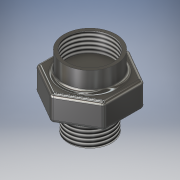
# Autodesk Inventor part: RKF 46-1M_NPT
Saved by Autodesk Inventor 2016 (Build 200138000, 138)
## iProperties
Created: 2016-03-26
Part Number: RKF 46-1M_NPT
Material: Brass, Soft Yellow
Document SubType Name: Modeling
Designer: agmle
Density: 8.47 g/cm^3
Appearance: Chrome - Polished
Author: agmle
Autodesk Inventor part; units mm, degrees
ref_plane "YZ Plane" through (0, 0, 0) normal (1, 0, 0) x (0, 1, 0)
ref_plane "XZ Plane" through (0, 0, 0) normal (0, 1, 0) x (-1, 0, 0)
ref_plane "XY Plane" through (0, 0, 0) normal (0, 0, 1) x (1, 0, 0)
sketch "Sketch1" plane through (0, 0, 0) normal (0, 1, 0) x (-1, 0, 0)
  line L0 (16.6553, -9.6469) -> (-0.0268, -19.2474)
  line L1 (-0.0268, -19.2474) -> (-16.6821, -9.6005)
  line L2 (-16.6821, -9.6005) -> (-16.6553, 9.6469)
  line L3 (-16.6553, 9.6469) -> (0.0268, 19.2474)
  line L4 (0.0268, 19.2474) -> (16.6821, 9.6005)
  line L5 (16.6821, 9.6005) -> (16.6553, -9.6469)
  point P0 (0, 0)
  point P1 (0, 0)
  dimension "d0" = 33.3375
  constraints: 12 end point, 1 coincident, 13 other
  measures "d0" distance between parallel lines of L2 L5
extrude "Extrusion1" add sketch "Sketch1" along normal blind 12.3031
sketch "Sketch2" plane through (0, 12.3031, 0) normal (0, 1, 0) x (1, 0, 0)
  circle A0 centre (0, 0) radius 12.7
  circle A1 centre (0, 0) radius 11.1125
  dimension "d3" = 25.4
  dimension "d16" = 22.225
  constraints: 2 centre point, 2 coincident
  measures "d3" diameter of A0
  measures "d16" diameter of A1
sketch "Sketch3" plane through (0, 0, 0) normal (0, -1, 0) x (1, 0, 0)
  circle A0 centre (0, 0) radius 10.541
  dimension "d8" = 21.082
  constraints: 1 centre point, 1 coincident
  measures "d8" diameter of A0
extrude "Extrusion3" add sketch "Sketch3" along normal blind 12.7
thread "Thread2" size "1/2" designation "1/2 - 14 NPT" standard "NPT" length 19.8628
fillet "Fillet1" radius 1.5875 6 edges at (16.6553, 6.1516, 9.6469) (-0.0268, 6.1516, 19.2474) (-16.6821, 6.1516, 9.6005) (16.6821, 6.1516, -9.6005) (0.0268, 6.1516, -19.2474) (-16.6553, 6.1516, -9.6469)
fillet "Fillet2" radius 1.5875 24 edges at (-16.4428, 12.3031, -9.5238) (-16.6687, 12.3031, -0.0232) (-16.4693, 12.3031, 9.478) (-8.3545, 12.3031, 14.4239) (-0.0265, 12.3031, 19.0018) (8.3143, 12.3031, 14.4471) (16.4428, 12.3031, 9.5238) (16.6687, 12.3031, 0.0232) (16.4693, 12.3031, -9.478) (8.3545, 12.3031, -14.4239) (0.0265, 12.3031, -19.0018) (-8.3143, 12.3031, -14.4471) (0.0265, 0, -19.0018) (8.3545, 0, -14.4239) (16.4693, 0, -9.478) (16.6687, 0, 0.0232) (16.4428, 0, 9.5238) (8.3143, 0, 14.4471) (-0.0265, 0, 19.0018) (-8.3545, 0, 14.4239) (-16.4693, 0, 9.478) (-16.6687, 0, -0.0232) (-16.4428, 0, -9.5238) (-8.3143, 0, -14.4471)
extrude "Extrusion4" add sketch "Sketch2" along normal blind 9.525
thread "Thread3" size "7/8-14 UNF" class "2B" standard "ANSI Unified Screw Threads" full length
fillet "Fillet4" radius 1.5875 1 edges at (-12.7, 12.3031, 0)
body "Solid1"
